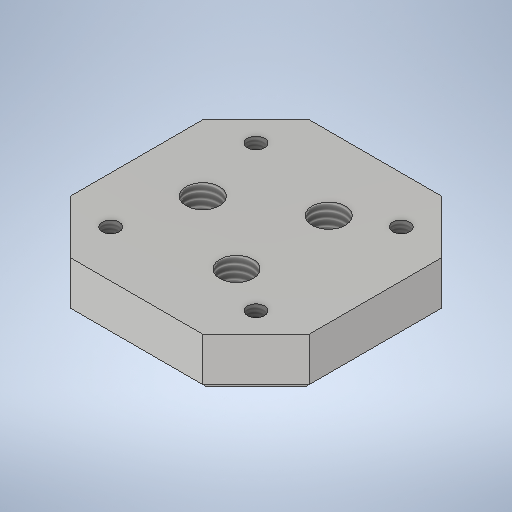
# Autodesk Inventor part: Platform B
Saved by Autodesk Inventor 2025 (Build 290162000, 162)
## iProperties
Created: 2021-01-07
Part Number: Platform B
Material: Generic
Document SubType Name: Modeling
Designer: caleb
Density: 1 g/cm^3
Appearance: Default
Mass: 4.3222 g
Surface Area: 23.732 cm^2
Volume: 4.3222 cm^3
Author: caleb
Autodesk Inventor part; units mm, degrees
ref_plane "YZ Plane" through (0, 0, 0) normal (1, 0, 0) x (0, 1, 0)
ref_plane "XZ Plane" through (0, 0, 0) normal (0, 1, 0) x (-1, 0, 0)
ref_plane "XY Plane" through (0, 0, 0) normal (0, 0, 1) x (1, 0, 0)
sketch "Sketch1" plane through (0, 0, 0) normal (0, 1, 0) x (-1, 0, 0)
  line L0 (-14.25, 14.25) -> (14.25, 14.25)
  line L1 (14.25, 14.25) -> (14.25, -14.25)
  line L2 (14.25, -14.25) -> (-14.25, -14.25)
  line L3 (-14.25, -14.25) -> (-14.25, 14.25)
  line L4 (-14.25, 14.25) -> (14.25, -14.25) construction
  line L5 (14.25, 14.25) -> (-14.25, -14.25) construction
  point P0 (0, 0)
  dimension "d0" = 28.5
  dimension "d1" = 28.5
  constraints: 12 end point, 2 midpoint, 2 parallel, 1 horizontal, 1 perpendicular
  measures "d0" distance of L0.end L1.end
  measures "d1" distance of L0.start L0.end
extrude "Extrusion1" add sketch "Sketch1" along normal blind 6
sketch "Sketch6" plane through (0, 0, 0) normal (0, -1, 0) x (1, 0, 0)
  point P0 (0, 0)
  point P1 (-6.35, 0)
  point P2 (3.175, -5.4993)
  point P3 (3.175, 5.4993)
  dimension "d77" = 6.35
  dimension "d93" = 360
  constraints: 1 horizontal alignment, 4 other
  measures "d77" distance of point (0, 0) point (-6.35, 0)
sketch "Sketch7" plane through (0, 6, 0) normal (0, 1, 0) x (1, 0, 0)
  circle A0 centre (0, 0) radius 12.25
  line L0 (0, 0) -> (-8.6621, -8.6621) construction
  line L1 (-8.6621, -8.6621) -> (-0.015, -8.6621) construction
  line L2 (-14.25, -14.25) -> (14.25, -14.25) construction
  line L3 (14.25, 14.25) -> (-14.25, 14.25) construction
  line L4 (14.25, -14.25) -> (14.25, 14.25) construction
  point P0 (8.6621, -8.6621)
  point P1 (8.6621, 8.6621)
  point P2 (-8.6621, 8.6621)
  dimension "d95" = 24.5
  dimension "d96" = 45
  dimension "d97" = 28.5
  dimension "d98" = 28.5
  dimension "d99" = 14.25
  dimension "d100" = 14.25
  dimension "d103" = 360
  constraints: 4 end point, 1 coincident, 1 horizontal, 8 other
  measures "d96" angle of L1 L0
  measures "d97" distance between parallel lines of L2 L3
  measures "d98" distance of L2.start L2.end
  measures "d99" distance from line of L4 L0.start
  measures "d100" distance from line of L2 L0.start
hole "Hole4" at (-8.6621, 6, -8.6621) at (-8.6621, 6, 8.6621) at (8.6621, 6, 8.6621) at (8.6621, 6, -8.6621) direction (0, -1, 0) diameter 2.013 depth 7.6 tip angle 118 thread size "M2.5x0.45" class "6H" standard "ANSI Metric M Profile"
hole "Hole5" at (-6.35, 0, 0) at (3.175, 0, -5.4993) at (3.175, 0, 5.4993) direction (0, 1, 0) diameter 3.9624 end through all thread size "10-32 UNF" class "2B" standard "ANSI Unified Screw Threads"
chamfer "Chamfer3" distance 6.35 angle 45 4 edges at (-14.25, 3, 14.25) (14.25, 3, 14.25) (14.25, 3, -14.25) (-14.25, 3, -14.25)
chamfer "Chamfer4" distance 0.7937 angle 45 8 edges at (0, 0, -14.25) (11.075, 0, -11.075) (14.25, 0, 0) (11.075, 0, 11.075) (0, 0, 14.25) (-11.075, 0, 11.075) (-14.25, 0, 0) (-11.075, 0, -11.075)
equation "\"d99\" = 0.5 * d98"
equation "\"d100\" = 0.5 * d97"
body "Solid1"
